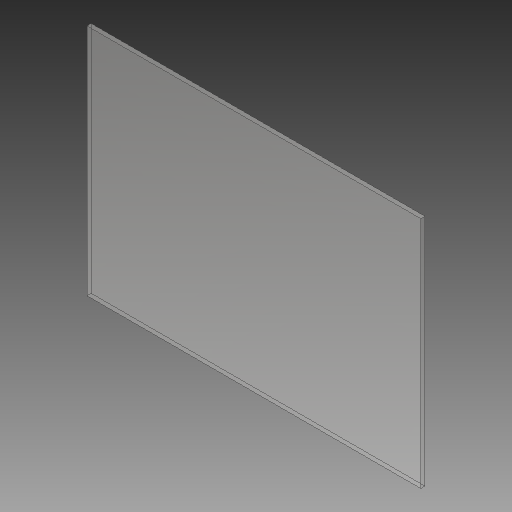
# Autodesk Inventor part: rest plate
Saved by Autodesk Inventor 2017 SP1 (Build 210196100, 196)
## iProperties
Created: 2018-01-26
Part Number: rest plate
Material: Polycarbonate, Clear
Document SubType Name: Modeling
Designer: Ben
Density: 1.2 g/cm^3
Appearance: Polycarbonate - Clear
Mass: 172.064 g
Surface Area: 930.643 cm^2
Volume: 143.387 cm^3
Author: Ben
Autodesk Inventor part; units mm, degrees
ref_plane "YZ Plane" through (0, 0, 0) normal (1, 0, 0) x (0, 1, 0)
ref_plane "XZ Plane" through (0, 0, 0) normal (0, 1, 0) x (-1, 0, 0)
ref_plane "XY Plane" through (0, 0, 0) normal (0, 0, 1) x (1, 0, 0)
sketch "Sketch1" plane through (0, 0, 0) normal (0, 0, 1) x (1, 0, 0)
  line L0 (-127, -88.9) -> (127, -88.9)
  line L1 (127, -88.9) -> (127, 88.9)
  line L2 (127, 88.9) -> (-127, 88.9)
  line L3 (-127, 88.9) -> (-127, -88.9)
  line L4 (-127, -88.9) -> (127, 88.9) construction
  line L5 (127, -88.9) -> (-127, 88.9) construction
  point P0 (0, 0)
  dimension "d0" = 254
  dimension "d1" = 177.8
  constraints: 12 end point, 2 midpoint, 2 parallel, 1 horizontal, 1 perpendicular
  measures "d0" distance of L1.end L2.end
  measures "d1" distance of L0.end L1.end
extrude "Extrusion1" add sketch "Sketch1" along normal blind 3.175
body "Solid1"
